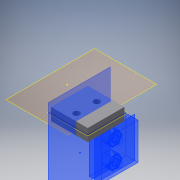
# Autodesk Inventor part: holder
Saved by Autodesk Inventor 2016 (Build 200138000, 138)
## iProperties
Created: 2016-01-21
Part Number: holder
Material: Generic
Document SubType Name: Modeling
Designer: Erwin Ried
Density: 1 g/cm^3
Appearance: Default
Author: Erwin Ried
Autodesk Inventor part; units mm, degrees
ref_plane "YZ Plane" through (0, 0, 0) normal (1, 0, 0) x (0, 1, 0)
ref_plane "XZ Plane" through (0, 0, 0) normal (0, 1, 0) x (-1, 0, 0)
ref_plane "XY Plane" through (0, 0, 0) normal (0, 0, 1) x (1, 0, 0)
ref_plane "Work Plane1" through (0, 0, 0) normal (0, 0, 1) x (1, 0, 0)
sketch "Sketch1" plane through (0, 0, 0) normal (0, 0, 1) x (1, 0, 0)
  arc A0 (-10.7354, 13.2764) -> (-8.7899, 5.3181) centre (6.5146, 13.2764) ccw projected
  line L0 (2.2646, -15.9406) -> (-8.7899, 5.3181) projected
  line L1 (2.2646, -15.9406) -> (17.0046, -15.9406) projected
  line L2 (17.0046, -15.9406) -> (17.0046, -1.0343) projected
  arc A1 (-5.2391, 19.424) -> (17.0046, -1.0343) centre (26.9358, 32.085) ccw projected
  arc A2 (-5.2391, 19.424) -> (-10.7354, 23.5341) centre (-10.7011, 17.8498) ccw projected
  line L3 (-10.7354, 23.5341) -> (-10.7354, 13.2764) projected
  line L4 (17.0046, -15.9406) -> (26.0046, -15.9406)
  line L5 (26.0046, -15.9406) -> (26.0046, 2.0594)
  line L6 (26.0046, 2.0594) -> (17.0046, 2.0594)
  line L7 (17.0046, 2.0594) -> (17.0046, -15.9406)
  line L8 (17.0046, -15.9406) -> (8.0046, -15.9406)
  line L9 (8.0046, -15.9406) -> (8.0046, 2.0594)
  line L10 (8.0046, 2.0594) -> (17.0046, 2.0594)
  line L11 (17.0046, 2.0594) -> (17.0046, -15.9406)
  point P0 (0, 0)
  dimension "d0" = 9
  dimension "d1" = 18
  dimension "d2" = 9
  constraints: 16 end point, 4 parallel, 2 horizontal, 2 perpendicular, 1 point on line
  measures "d0" distance of L6.end L5.end
  measures "d1" distance of L5.end L4.end
  measures "d2" distance of L9.end L10.end
extrude "Extrusion1" add sketch "Sketch1" along normal blind 6 contours L9 L10 A1 L2 L1 | L10 L7 A1 | L2 L7 L6 L5 L4
sketch "Sketch2" plane through (0, 0, 6) normal (0, 0, 1) x (1, 0, 0)
  line L0 (26.0046, 2.0594) -> (8.0046, 2.0594) projected
  line L1 (8.0046, 2.0594) -> (8.0046, -15.9406) projected
  line L2 (8.0046, -15.9406) -> (26.0046, -15.9406) projected
  line L3 (26.0046, -15.9406) -> (26.0046, 2.0594) projected
  line L4 (17.0046, -15.9406) -> (17.0046, -12.4406) construction
  line L5 (17.0046, -12.4406) -> (17.0046, -2.4406) construction
  point P0 (0, 0)
  dimension "d5" = 3.5
  dimension "d6" = 10
  constraints: 4 end point, 1 midpoint, 1 point on line, 1 vertical
  measures "d5" distance of L4.start L4.end
  measures "d6" distance of L4.end L5.end
hole "Hole1" at (17.0046, -12.4406, 6) at (17.0046, -2.4406, 6) direction (0, 0, -1) diameter 3 end through all
sketch "Sketch3" plane through (0, 0, 0) normal (0, 0, -1) x (-1, 0, 0)
  circle A0 centre (-17.0046, -12.4406) radius 1.5 projected
  circle A1 centre (-17.0046, -2.4406) radius 1.5 projected
  line L0 (-8.0046, -15.9406) -> (-26.0046, -15.9406) projected
  line L1 (-8.0046, 2.0594) -> (-8.0046, -15.9406) projected
  line L2 (-26.0046, 2.0594) -> (-8.0046, 2.0594) projected
  line L3 (-26.0046, -15.9406) -> (-26.0046, 2.0594) projected
  line L4 (-20.2955, -12.4406) -> (-18.65, -9.5906)
  line L5 (-18.65, -9.5906) -> (-15.3591, -9.5906)
  line L6 (-15.3591, -9.5906) -> (-13.7137, -12.4406)
  line L7 (-13.7137, -12.4406) -> (-15.3591, -15.2906)
  line L8 (-15.3591, -15.2906) -> (-18.65, -15.2906)
  line L9 (-18.65, -15.2906) -> (-20.2955, -12.4406)
  line L10 (-20.2955, -2.4406) -> (-18.65, 0.4094)
  line L11 (-18.65, 0.4094) -> (-15.3591, 0.4094)
  line L12 (-15.3591, 0.4094) -> (-13.7137, -2.4406)
  line L13 (-13.7137, -2.4406) -> (-15.3591, -5.2906)
  line L14 (-15.3591, -5.2906) -> (-18.65, -5.2906)
  line L15 (-18.65, -5.2906) -> (-20.2955, -2.4406)
  point P0 (0, 0)
  dimension "d14" = 5.7
  constraints: 24 end point, 2 coincident, 26 other
  measures "d14" distance between parallel lines of L7 L4
ref_plane "Work Plane2" through (0, 0, 3.5) normal (0, 0, -1) x (-1, 0, 0)
sketch "Sketch4" plane through (0, 0, 3.5) normal (0, 0, -1) x (-1, 0, 0)
  line L0 (-18.65, 0.4094) -> (-15.3591, 0.4094) projected
  line L1 (-20.2955, -2.4406) -> (-18.65, 0.4094) projected
  circle A0 centre (-17.0046, -2.4406) radius 1.5 projected
  circle A1 centre (-17.0046, -12.4406) radius 1.5 projected
  line L2 (-15.3591, -5.2906) -> (-18.65, -5.2906) projected
  line L3 (-18.65, -9.5906) -> (-15.3591, -9.5906) projected
  line L4 (-20.2955, -12.4406) -> (-18.65, -9.5906) projected
  line L5 (-20.2955, -12.4406) -> (-18.65, -9.5906)
  line L6 (-18.65, -9.5906) -> (-15.3591, -9.5906)
  line L7 (-15.3591, -9.5906) -> (-13.7137, -12.4406)
  line L8 (-13.7137, -12.4406) -> (-15.3591, -15.2906)
  line L9 (-15.3591, -15.2906) -> (-18.65, -15.2906)
  line L10 (-18.65, -15.2906) -> (-20.2955, -12.4406)
  line L11 (-20.2955, -2.4406) -> (-18.65, 0.4094)
  line L12 (-18.65, 0.4094) -> (-15.3591, 0.4094)
  line L13 (-15.3591, 0.4094) -> (-13.7137, -2.4406)
  line L14 (-13.7137, -2.4406) -> (-15.3591, -5.2906)
  line L15 (-15.3591, -5.2906) -> (-18.65, -5.2906)
  line L16 (-18.65, -5.2906) -> (-20.2955, -2.4406)
  point P0 (0, 0)
  constraints: 24 end point, 2 coincident, 26 other
extrude "Extrusion2" cut sketch "Sketch3" against normal blind 4 contours L4 L5 L6 L7 L8 L9 | L10 L11 L12 L13 L14 L15
body "Solid1"
